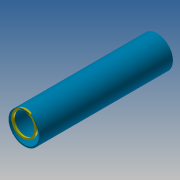
# Autodesk Inventor part: 2h2slv
Saved by Autodesk Inventor 2014 SP1 (Build 180222100, 222)
## iProperties
Company: HERA Project
Created: 2013-05-14
Part Number: 2h2slv
Material: PVC-Piping
Document SubType Name: Modeling
Designer: David DeBoer
Density: 1.4 g/cm^3
Mass: 429.807 g
Surface Area: 1214.86 cm^2
Volume: 307.005 cm^3
Description: Hub mating sleeve
Appearance: Smooth - White
Author: David DeBoer
Title: Hub mating sleeve
Autodesk Inventor part; units mm, degrees
ref_plane "YZ Plane" through (0, 0, 0) normal (1, 0, 0) x (0, 1, 0)
ref_plane "XZ Plane" through (0, 0, 0) normal (0, 1, 0) x (-1, 0, 0)
ref_plane "XY Plane" through (0, 0, 0) normal (0, 0, 1) x (1, 0, 0)
sketch "Sketch1" plane through (0, 0, 0) normal (0, 0, 1) x (1, 0, 0)
  circle A0 centre (0, 0) radius 45
  circle A1 centre (0, 0) radius 41.1
  dimension "d0" = 90
  dimension "d2" = 3.9
  constraints: 2 centre point, 1 coincident
  measures "d0" diameter of A0
  measures "d2" radial gap between concentric circles of A1 A0
extrude "Extrusion1" add sketch "Sketch1" along normal blind 377
sketch "Sketch2" plane through (0, 0, 377) normal (0, 0, 1) x (1, 0, 0)
  circle A0 centre (0, 0) radius 41.1 projected
  circle A1 centre (0, 0) radius 45 projected
  point P0 (0, 45)
  constraints: 1 vertical alignment, 1 other
ref_plane "Work Plane1" through (0, 45, 377) normal (0, 1, 0) x (-1, 0, 0)
sketch "Sketch5" plane through (0, 45, 377) normal (0, 1, 0) x (-1, 0, 0)
  circle A0 centre (0, -357) radius 4.4901
  point P0 (0, -377)
  dimension "d25" = 20
  constraints: 1 centre point
  measures "d25" distance of point (0, -377) A0.centre
hole "nailHole" at (0, 45, 20) direction (0, -1, 0) diameter 3.175 end through all
sketch "Sketch6" plane through (0, 0, 377) normal (0, 0, 1) x (1, 0, 0)
  circle A0 centre (0, 0) radius 41.1 projected
  circle A1 centre (0, 0) radius 45 projected
  point P0 (0, 45)
  constraints: 1 vertical alignment, 1 other
ref_plane "Work Plane2" through (0, 45, 377) normal (0, 1, 0) x (-1, 0, 0)
sketch "Sketch10" plane through (0, 0, 377) normal (0, 0, 1) x (1, 0, 0)
  circle A0 centre (0, 0) radius 41.1 projected
  circle A1 centre (0, 0) radius 45 projected
  line L0 (0, 41.1) -> (46.8002, 41.1) construction
  constraints: 2 end point, 2 horizontal, 1 vertical alignment, 1 other
ref_plane "Work Plane3" through (0, 41.1, 377) normal (0, 0.0650548, 0.9978817) x (1, 0, 0)
sketch "Sketch11" plane through (0, 41.1, 377) normal (0, 0.0650548, 0.9978817) x (1, 0, 0)
  circle A0 centre (0, -30.1983) radius 30.1625
  circle A1 centre (0, -30.1983) radius 35.2425
  point P0 (0, -16.4873)
  dimension "d44" = 60.325
  dimension "d45" = 5.08
  constraints: 2 centre point
  measures "d44" diameter of A0
  measures "d45" radial gap between concentric circles of A0 A1
extrude "INSERT_GUIDE_NOTFAB" add sketch "Sketch11" against normal blind 5.08
sketch "Sketch12" plane through (0, 41.1, 377) normal (0, 0.0650548, 0.9978817) x (1, 0, 0)
  circle A0 centre (0, -30.1983) radius 30.1625 projected
  line L0 (-1.27, -0.4213) -> (1.27, -0.4213)
  line L1 (1.27, -0.4213) -> (1.27, 2.1187)
  line L2 (1.27, 2.1187) -> (-1.27, 2.1187)
  line L3 (-1.27, 2.1187) -> (-1.27, -0.4213)
  line L4 (0, 2.1187) -> (0, -0.4213) construction
  line L5 (0, -16.4873) -> (0, -30.1983) construction
  dimension "d48" = 2.54
  dimension "d49" = 2.54
  constraints: 12 end point, 2 collinear, 2 midpoint, 2 parallel, 1 horizontal, 1 perpendicular
  measures "d48" distance of L2.end L1.end
  measures "d49" distance of L1.end L0.end
extrude "INSERT_KEY_NOTFAB" cut sketch "Sketch12" along normal mid plane 12.7 contours L1 L0 L3 A0 | A0 L3 L2 L1 picked at (0.1411, -0.2938)
equation "\"d0\" = sleeveOD"
equation "\"d2\" = sleeveWall"
equation "\"d3\" = sleeveLength"
equation "\"d25\" = nailDelta"
equation "\"sleeveOD\" = 90"
equation "\"sleeveWall\" = 3.9"
equation "\"sleeveLength\" = 377"
equation "\"nailDelta\" = 20"
equation "\"sparLaunchAngle\" = 3.72deg"
body "Solid1"
